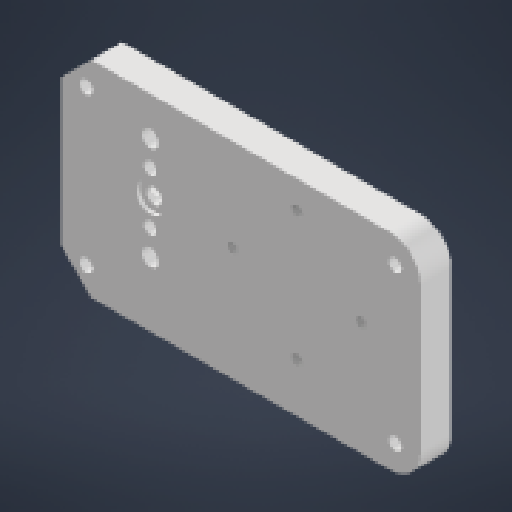
# Autodesk Inventor part: Base
Saved by Autodesk Inventor 2025.4 (Build 294407000, 407)
## iProperties
Created: 2026-05-29
Part Number: Base
Material: Generic
Document SubType Name: Modeling
Designer: VuQuan
Density: 1 g/cm^3
Appearance: Default
Author: VuQuan
Autodesk Inventor part; units mm, degrees
ref_plane "YZ Plane" through (0, 0, 0) normal (1, 0, 0) x (0, 1, 0)
ref_plane "XZ Plane" through (0, 0, 0) normal (0, 1, 0) x (-1, 0, 0)
ref_plane "XY Plane" through (0, 0, 0) normal (0, 0, 1) x (1, 0, 0)
sketch "Sketch1" plane through (0, 0, 0) normal (0, 0, 1) x (1, 0, 0)
  line L0 (-58, 40) -> (58, 40)
  line L1 (70, 28) -> (70, -28)
  line L2 (58, -40) -> (-58, -40)
  line L3 (-70, -28) -> (-70, 28)
  arc A0 (70, 28) -> (58, 40) centre (58, 28) ccw
  arc A1 (58, -40) -> (70, -28) centre (58, -28) ccw
  line L4 (-58, 40) -> (-70, 28)
  line L5 (-70, -28) -> (-58, -40)
  line L6 (-70, 0) -> (70, 0) construction
  circle A2 centre (-60, 30) radius 2.6
  circle A3 centre (60, 30) radius 2.6
  line L7 (66.4853, 36.4853) -> (58, 28) construction
  circle A4 centre (-60, -30) radius 2.6
  circle A5 centre (60, -30) radius 2.6
  point P0 (0, 0)
  point P1 (-70, 40)
  point P2 (-70, -40)
  point P3 (0, 40)
  dimension "d0" = 140
  dimension "d1" = 80
  dimension "d2" = 12
  dimension "d3" = 12
  dimension "d4" = 12
  dimension "d5" = 12
  dimension "d6" = 12
  dimension "d7" = 5.2
  dimension "d8" = 120
  dimension "d9" = 60
  constraints: 16 end point, 6 centre point, 5 point on circle, 5 point on line, 4 tangent, 3 midpoint, 2 equal radius, 2 horizontal alignment, 2 parallel, 2 symmetric about line, 1 horizontal, 1 perpendicular, 1 vertical alignment, 2 other
  measures "d0" distance between parallel lines of L1 L3
  measures "d1" distance between parallel lines of L2 L0
  measures "d2" radius of A0
  measures "d3" distance of L0.start point (-70, 40)
  measures "d4" distance of L3.end point (-70, 40)
  measures "d5" distance of L3.start point (-70, -40)
  measures "d6" distance of L2.end point (-70, -40)
  measures "d7" diameter of A3
  measures "d8" distance of A3.centre A2.centre
  measures "d9" diameter of A3.centre L6
extrude "Extrusion1" add sketch "Sketch1" along normal mid plane 12
sketch "Sketch2" plane through (-70, -28, 6) normal (-1, 0, 0) x (0, 0, 1)
  line L0 (-12, 68) -> (0, 68) projected
  point P0 (-6, 28)
  point P1 (-6, 33)
  dimension "d12" = 35
  constraints: 1 vertical alignment
  measures "d12" distance from line of L0 point (-6, 33)
hole "Hole1" at (-70, 5, 0) direction (1, 0, 0) diameter 6 depth 88 tip angle 118
sketch "Sketch3" plane through (0, 0, 6) normal (0, 0, 1) x (1, 0, 0)
  line L0 (70, -28) -> (70, 28) projected
  line L1 (-70, 28) -> (-70, -28) projected
  circle A0 centre (22, 4) radius 25 construction
  line L2 (-70, 2) -> (-70, 8) projected
  line L3 (-70, 2) -> (-70, 8) projected
  line L4 (18, 8) -> (18, 2) projected
  line L5 (18, 5) -> (-70, 5) construction
  circle A1 centre (-35, 5) radius 5.5
  circle A2 centre (-35, 25) radius 5.5
  circle A3 centre (-35, 25) radius 3.25
  circle A4 centre (-35, -15) radius 5.5
  circle A5 centre (-35, -15) radius 3.25
  circle A6 centre (-35, 15) radius 2.5
  circle A7 centre (-35, -5) radius 2.5
  circle A8 centre (-35, 5) radius 3
  line L6 (58, 40) -> (-58, 40) projected
  point P0 (0, 0)
  point P1 (22, 29)
  point P2 (-3, 4)
  point P3 (22, -21)
  point P4 (47, 4)
  dimension "d22" = 50
  dimension "d20" = 48
  dimension "d25" = 360
  dimension "d27" = 11
  dimension "d28" = 35
  dimension "d30" = 11
  dimension "d31" = 6.5
  dimension "d32" = 20
  dimension "d33" = 5
  dimension "d34" = 10
  dimension "d51" = 6
  dimension "d59" = 36
  constraints: 8 centre point, 4 vertical alignment, 3 coincident, 3 symmetric about line, 2 end point, 2 midpoint, 1 point on line, 10 other
  measures "d20" distance from line of L0 point (22, 4)
  measures "d27" diameter of A1
  measures "d28" distance from line of L1 A1.centre
  measures "d30" diameter of A2
  measures "d31" diameter of A3
  measures "d32" distance of A2.centre A1.centre
  measures "d33" diameter of A6
  measures "d34" distance of A1.centre A6.centre
  measures "d51" diameter of A8
  measures "d59" distance from line of L6 point (22, 4)
hole "Hole2" at (22, 29, 6) at (47, 4, 6) at (22, -21, 6) at (-3, 4, 6) direction (0, 0, -1) diameter 4.134 depth 12 thread size "M5x0.8" class "6H" standard "ISO Metric profile"
extrude "Extrusion2" cut sketch "Sketch3" against normal through all contours A3 | A5 | A6 | A7
extrude "Extrusion3" cut sketch "Sketch3" along normal blind 6 from surface at -12 contours A2 | A4
extrude "Extrusion4" cut sketch "Sketch3" against normal blind 1.5 contours A1 | A8
extrude "Extrusion5" cut sketch "Sketch3" against normal up to surface contours A8
sketch "Sketch4" plane through (-70, -28, 6) normal (-1, 0, 0) x (0, 0, 1)
  circle A0 centre (-6, 33) radius 3 projected
  point P0 (-6, 28)
  constraints: 1 coincident
hole "Hole3" at (-70, 5, 0) direction (1, 0, 0) diameter 6.647 depth 15 thread size "M8x1.25" class "6H" standard "ISO Metric profile"
equation "\"d4\" = d3"
equation "\"d5\" = d3"
equation "\"d6\" = d5"
body "Solid1"
